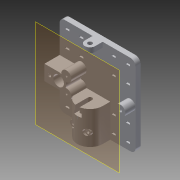
# Autodesk Inventor part: EFFECTOR SECONDARY PLATE
Saved by Autodesk Inventor 2013 (Build 170138000, 138)
## iProperties
Created: 2014-03-03
Part Number: EFFECTOR SECONDARY PLATE
Material: Generic
Document SubType Name: Modeling
Designer: employee
Density: 1 g/cm^3
Author: employee
Autodesk Inventor part; units mm, degrees
ref_plane "YZ Plane" through (0, 0, 0) normal (1, 0, 0) x (0, 1, 0)
ref_plane "XZ Plane" through (0, 0, 0) normal (0, 1, 0) x (-1, 0, 0)
ref_plane "XY Plane" through (0, 0, 0) normal (0, 0, 1) x (1, 0, 0)
sketch "Sketch1" plane through (0, 0, 0) normal (0, 0, 1) x (1, 0, 0)
  arc A0 (-32.5, 40) -> (-37.5, 35) centre (-32.5, 35) ccw projected
  line L0 (-37.5, 35) -> (-37.5, 12.5) projected
  arc A1 (-37.5, -35) -> (-32.5, -40) centre (-32.5, -35) ccw projected
  line L1 (-32.5, -40) -> (32.5, -40) projected
  arc A2 (32.5, -40) -> (37.5, -35) centre (32.5, -35) ccw projected
  line L2 (37.5, -35) -> (37.5, -12.5) projected
  arc A3 (37.5, 35) -> (32.5, 40) centre (32.5, 35) ccw projected
  line L3 (32.5, 40) -> (-32.5, 40) projected
  line L4 (-18, -34) -> (-18, -32.5) projected
  line L5 (-18, -32.5) -> (-14, -32.5) projected
  line L6 (-14, -32.5) -> (-14, -34) projected
  line L7 (-14, -34) -> (-18, -34) projected
  line L8 (-32, -16) -> (-28, -16) projected
  line L9 (-28, -16) -> (-28, -17.5) projected
  line L10 (-28, -17.5) -> (-32, -17.5) projected
  line L11 (-32, -17.5) -> (-32, -16) projected
  line L12 (-14, -16) -> (-14, -17.5) projected
  line L13 (-14, -17.5) -> (-18, -17.5) projected
  line L14 (-18, -17.5) -> (-18, -16) projected
  line L15 (-18, -16) -> (-14, -16) projected
  line L16 (-28, -34) -> (-32, -34) projected
  line L17 (-32, -34) -> (-32, -32.5) projected
  line L18 (-32, -32.5) -> (-28, -32.5) projected
  line L19 (-28, -32.5) -> (-28, -34) projected
  line L20 (18, -32.5) -> (18, -34) projected
  line L21 (18, -34) -> (14, -34) projected
  line L22 (14, -34) -> (14, -32.5) projected
  line L23 (14, -32.5) -> (18, -32.5) projected
  line L24 (28, -16) -> (32, -16) projected
  line L25 (32, -16) -> (32, -17.5) projected
  line L26 (32, -17.5) -> (28, -17.5) projected
  line L27 (28, -17.5) -> (28, -16) projected
  line L28 (14, -17.5) -> (14, -16) projected
  line L29 (14, -16) -> (18, -16) projected
  line L30 (18, -16) -> (18, -17.5) projected
  line L31 (18, -17.5) -> (14, -17.5) projected
  line L32 (32, -34) -> (28, -34) projected
  line L33 (28, -34) -> (28, -32.5) projected
  line L34 (28, -32.5) -> (32, -32.5) projected
  line L35 (32, -32.5) -> (32, -34) projected
  line L36 (-18, 32.5) -> (-18, 34) projected
  line L37 (-18, 34) -> (-14, 34) projected
  line L38 (-14, 34) -> (-14, 32.5) projected
  line L39 (-14, 32.5) -> (-18, 32.5) projected
  line L40 (-28, 16) -> (-32, 16) projected
  line L41 (-32, 16) -> (-32, 17.5) projected
  line L42 (-32, 17.5) -> (-28, 17.5) projected
  line L43 (-28, 17.5) -> (-28, 16) projected
  line L44 (-14, 17.5) -> (-14, 16) projected
  line L45 (-14, 16) -> (-18, 16) projected
  line L46 (-18, 16) -> (-18, 17.5) projected
  line L47 (-18, 17.5) -> (-14, 17.5) projected
  line L48 (-32, 34) -> (-28, 34) projected
  line L49 (-28, 34) -> (-28, 32.5) projected
  line L50 (-28, 32.5) -> (-32, 32.5) projected
  line L51 (-32, 32.5) -> (-32, 34) projected
  line L52 (14, 32.5) -> (14, 34) projected
  line L53 (14, 34) -> (18, 34) projected
  line L54 (18, 34) -> (18, 32.5) projected
  line L55 (18, 32.5) -> (14, 32.5) projected
  line L56 (28, 32.5) -> (28, 34) projected
  line L57 (28, 34) -> (32, 34) projected
  line L58 (32, 34) -> (32, 32.5) projected
  line L59 (32, 32.5) -> (28, 32.5) projected
  line L60 (18, 17.5) -> (18, 16) projected
  line L61 (18, 16) -> (14, 16) projected
  line L62 (14, 16) -> (14, 17.5) projected
  line L63 (14, 17.5) -> (18, 17.5) projected
  line L64 (32, 17.5) -> (32, 16) projected
  line L65 (32, 16) -> (28, 16) projected
  line L66 (28, 16) -> (28, 17.5) projected
  line L67 (28, 17.5) -> (32, 17.5) projected
  arc A4 (-32.5, -7.5) -> (-37.5, -12.5) centre (-32.5, -12.5) ccw projected
  line L68 (-37.5, -12.5) -> (-37.5, -35) projected
  arc A5 (37.5, -12.5) -> (32.5, -7.5) centre (32.5, -12.5) ccw projected
  line L69 (32.5, -7.5) -> (22.5, -7.5) projected
  arc A6 (22.5, 7.5) -> (22.5, -7.5) centre (22.5, 0) ccw projected
  line L70 (22.5, 7.5) -> (32.5, 7.5) projected
  arc A7 (32.5, 7.5) -> (37.5, 12.5) centre (32.5, 12.5) ccw projected
  line L71 (37.5, 12.5) -> (37.5, 35) projected
  arc A8 (-37.5, 12.5) -> (-32.5, 7.5) centre (-32.5, 12.5) ccw projected
  line L72 (-32.5, 7.5) -> (-22.5, 7.5) projected
  arc A9 (-22.5, -7.5) -> (-22.5, 7.5) centre (-22.5, 0) ccw projected
  line L73 (-22.5, -7.5) -> (-32.5, -7.5) projected
  point P0 (0, 0)
extrude "Extrusion1" add sketch "Sketch1" along normal blind 5
sketch "Sketch2" plane through (-32.5, -40, 0) normal (0, -1, 0) x (1, 0, 0)
  line L0 (65, 0) -> (0, 0) projected
  line L1 (0, 0) -> (0, 5) projected
  line L2 (20, 0) -> (20, 12.5)
  arc A0 (45, 12.5) -> (20, 12.5) centre (32.5, 12.5) ccw
  line L3 (45, 12.5) -> (45, 0)
  point P0 (32.5, 0)
  point P1 (32.5, 0)
  dimension "d2" = 12.5
  dimension "d3" = 12.5
  constraints: 4 end point, 2 point on circle, 2 point on line, 2 tangent, 1 centre point, 1 midpoint, 1 parallel, 1 perpendicular, 1 vertical alignment
  measures "d2" distance from line of A0.centre L0
  measures "d3" radius of A0
extrude "Extrusion2" add sketch "Sketch2" against normal blind 19
sketch "Sketch3" plane through (-32.5, -40, 0) normal (0, -1, 0) x (1, 0, 0)
  arc A0 (45, 12.5) -> (20, 12.5) centre (32.5, 12.5) ccw projected
  circle A1 centre (32.5, 12.5) radius 8.1
  point P0 (32.5, 0)
  dimension "d6" = 16.2
  constraints: 1 centre point, 1 coincident
  measures "d6" diameter of A1
extrude "Extrusion3" cut sketch "Sketch3" against normal up to surface (19 mm away)
sketch "Sketch4" plane through (0, 0, 0) normal (0, 0, -1) x (-1, 0, 0)
  line L0 (-32.5, -40) -> (32.5, -40) projected
  line L1 (-28, 17.5) -> (-28, 16) projected
  line L2 (-7.25, -27.5) -> (7.25, -27.5)
  circle A0 centre (-7.25, -27.5) radius 1.5
  circle A1 centre (7.25, -27.5) radius 1.5
  point P0 (0, 0)
  point P1 (0, -40)
  point P2 (0, -27.5)
  dimension "d10" = 12.5
  dimension "d11" = 3
  dimension "d12" = 14.5
  constraints: 2 centre point, 2 coincident, 2 end point, 2 midpoint, 1 equal radius, 1 perpendicular, 1 vertical alignment
  measures "d10" distance between parallel lines of L0 L2
  measures "d11" diameter of A1
  measures "d12" distance of L2.start L2.end
extrude "Extrusion4" cut sketch "Sketch4" against normal through all
ref_plane "Work Plane1" through (0, 0, 25) normal (0, 0, 1) x (1, 0, 0)
sketch "Sketch5" plane through (0, 0, 25) normal (0, 0, 1) x (1, 0, 0)
  circle A0 centre (7.25, -27.5) radius 1.5 projected
  circle A1 centre (-7.25, -27.5) radius 1.5 projected
  line L0 (32.5, -40) -> (-32.5, -40) projected
  arc A2 (-37.5, -35) -> (-32.5, -40) centre (-32.5, -35) ccw projected
  line L1 (-37.5, 12.5) -> (-37.5, 35) projected
  arc A3 (-32.5, 40) -> (-37.5, 35) centre (-32.5, 35) ccw projected
  line L2 (-32.5, 40) -> (32.5, 40) projected
  arc A4 (37.5, 35) -> (32.5, 40) centre (32.5, 35) ccw projected
  line L3 (37.5, -12.5) -> (37.5, -35) projected
  arc A5 (32.5, -40) -> (37.5, -35) centre (32.5, -35) ccw projected
  line L4 (-14, -32.5) -> (-18, -32.5) projected
  line L5 (-18, -32.5) -> (-18, -34) projected
  line L6 (-18, -34) -> (-14, -34) projected
  line L7 (-14, -34) -> (-14, -32.5) projected
  line L8 (-28, -17.5) -> (-28, -16) projected
  line L9 (-28, -16) -> (-32, -16) projected
  line L10 (-32, -16) -> (-32, -17.5) projected
  line L11 (-32, -17.5) -> (-28, -17.5) projected
  line L12 (-18, -17.5) -> (-14, -17.5) projected
  line L13 (-14, -17.5) -> (-14, -16) projected
  line L14 (-14, -16) -> (-18, -16) projected
  line L15 (-18, -16) -> (-18, -17.5) projected
  line L16 (-32, -32.5) -> (-32, -34) projected
  line L17 (-32, -34) -> (-28, -34) projected
  line L18 (-28, -34) -> (-28, -32.5) projected
  line L19 (-28, -32.5) -> (-32, -32.5) projected
  line L20 (14, -34) -> (18, -34) projected
  line L21 (18, -34) -> (18, -32.5) projected
  line L22 (18, -32.5) -> (14, -32.5) projected
  line L23 (14, -32.5) -> (14, -34) projected
  line L24 (32, -17.5) -> (32, -16) projected
  line L25 (32, -16) -> (28, -16) projected
  line L26 (28, -16) -> (28, -17.5) projected
  line L27 (28, -17.5) -> (32, -17.5) projected
  line L28 (18, -16) -> (14, -16) projected
  line L29 (14, -16) -> (14, -17.5) projected
  line L30 (14, -17.5) -> (18, -17.5) projected
  line L31 (18, -17.5) -> (18, -16) projected
  line L32 (28, -32.5) -> (28, -34) projected
  line L33 (28, -34) -> (32, -34) projected
  line L34 (32, -34) -> (32, -32.5) projected
  line L35 (32, -32.5) -> (28, -32.5) projected
  line L36 (-14, 34) -> (-18, 34) projected
  line L37 (-18, 34) -> (-18, 32.5) projected
  line L38 (-18, 32.5) -> (-14, 32.5) projected
  line L39 (-14, 32.5) -> (-14, 34) projected
  line L40 (-32, 17.5) -> (-32, 16) projected
  line L41 (-32, 16) -> (-28, 16) projected
  line L42 (-28, 16) -> (-28, 17.5) projected
  line L43 (-28, 17.5) -> (-32, 17.5) projected
  line L44 (-18, 16) -> (-14, 16) projected
  line L45 (-14, 16) -> (-14, 17.5) projected
  line L46 (-14, 17.5) -> (-18, 17.5) projected
  line L47 (-18, 17.5) -> (-18, 16) projected
  line L48 (-28, 32.5) -> (-28, 34) projected
  line L49 (-28, 34) -> (-32, 34) projected
  line L50 (-32, 34) -> (-32, 32.5) projected
  line L51 (-32, 32.5) -> (-28, 32.5) projected
  line L52 (18, 34) -> (14, 34) projected
  line L53 (14, 34) -> (14, 32.5) projected
  line L54 (14, 32.5) -> (18, 32.5) projected
  line L55 (18, 32.5) -> (18, 34) projected
  line L56 (32, 34) -> (28, 34) projected
  line L57 (28, 34) -> (28, 32.5) projected
  line L58 (28, 32.5) -> (32, 32.5) projected
  line L59 (32, 32.5) -> (32, 34) projected
  line L60 (14, 16) -> (18, 16) projected
  line L61 (18, 16) -> (18, 17.5) projected
  line L62 (18, 17.5) -> (14, 17.5) projected
  line L63 (14, 17.5) -> (14, 16) projected
  line L64 (28, 16) -> (32, 16) projected
  line L65 (32, 16) -> (32, 17.5) projected
  line L66 (32, 17.5) -> (28, 17.5) projected
  line L67 (28, 17.5) -> (28, 16) projected
  circle A6 centre (-7.25, -27.5) radius 3
  circle A7 centre (7.25, -27.5) radius 3
  line L68 (-37.5, -35) -> (-37.5, -12.5) projected
  arc A8 (-32.5, -7.5) -> (-37.5, -12.5) centre (-32.5, -12.5) ccw projected
  line L69 (-32.5, -7.5) -> (-22.5, -7.5) projected
  arc A9 (-22.5, -7.5) -> (-22.5, 7.5) centre (-22.5, 0) ccw projected
  line L70 (-22.5, 7.5) -> (-32.5, 7.5) projected
  arc A10 (-37.5, 12.5) -> (-32.5, 7.5) centre (-32.5, 12.5) ccw projected
  line L71 (37.5, 35) -> (37.5, 12.5) projected
  arc A11 (32.5, 7.5) -> (37.5, 12.5) centre (32.5, 12.5) ccw projected
  line L72 (32.5, 7.5) -> (22.5, 7.5) projected
  arc A12 (22.5, 7.5) -> (22.5, -7.5) centre (22.5, 0) ccw projected
  line L73 (22.5, -7.5) -> (32.5, -7.5) projected
  arc A13 (37.5, -12.5) -> (32.5, -7.5) centre (32.5, -12.5) ccw projected
  point P0 (0, 0)
  dimension "d16" = 6
  constraints: 2 centre point, 2 coincident, 1 equal radius
  measures "d16" diameter of A7
extrude "Extrusion5" add sketch "Sketch5" against normal up to surface contours A6 | A7
sketch "Sketch6" plane through (-7.25, -27.5, 25) normal (0, 0, 1) x (1, 0, 0)
  circle A0 centre (0, 0) radius 1.5 projected
  circle A1 centre (0, 0) radius 3 projected
  circle A2 centre (14.5, 0) radius 1.5 projected
  circle A3 centre (14.5, 0) radius 3 projected
  point P0 (7.25, 27.5)
extrude "Extrusion6" cut sketch "Sketch6" against normal blind 3
sketch "Sketch7" plane through (-32.5, -21, 0) normal (0, 1, 0) x (1, 0, 0)
  arc A0 (29.4406, -5) -> (35.5594, -5) centre (32.5, -12.5) ccw projected
  line L0 (20, -5) -> (29.4406, -5) projected
  line L1 (20, -5) -> (20, -12.5) projected
  arc A1 (20, -12.5) -> (45, -12.5) centre (32.5, -12.5) ccw projected
  line L2 (45, -12.5) -> (45, -5) projected
  line L3 (35.5594, -5) -> (45, -5) projected
  line L4 (29.4406, -5) -> (35.5594, -5)
  circle A2 centre (32.5, -12.5) radius 1
  point P0 (32.5, 0)
  dimension "d22" = 2
  constraints: 2 end point, 1 centre point, 1 coincident, 1 collinear
  measures "d22" diameter of A2
extrude "Extrusion7" add sketch "Sketch7" along normal blind 5
fillet "Fillet1" radius 2 1 edges at (-1, -16, 12.5)
sketch "Sketch8" plane through (-32.5, -16, 0) normal (0, 1, 0) x (1, 0, 0)
  line L0 (20, -5) -> (45, -5) projected
  line L1 (20, -5) -> (20, -12.5) projected
  arc A0 (20, -12.5) -> (45, -12.5) centre (32.5, -12.5) ccw projected
  line L2 (45, -12.5) -> (45, -5) projected
  circle A1 centre (32.5, -12.5) radius 3 projected
  line L3 (32.5, -8.3431) -> (36.1, -10.4215)
  line L4 (36.1, -10.4215) -> (36.1, -14.5785)
  line L5 (36.1, -14.5785) -> (32.5, -16.6569)
  line L6 (32.5, -16.6569) -> (28.9, -14.5785)
  line L7 (28.9, -14.5785) -> (28.9, -10.4215)
  line L8 (28.9, -10.4215) -> (32.5, -8.3431)
  line L9 (28.9, -14.5785) -> (28.9, -24.4704)
  line L10 (36.1, -14.5785) -> (36.1, -24.4704)
  point P0 (32.5, 0)
  dimension "d28" = 7.2
  constraints: 16 end point, 2 point on circle, 1 coincident, 1 collinear, 1 parallel, 1 vertical, 13 other
  measures "d28" distance between parallel lines of L4 L7
extrude "Extrusion8" add sketch "Sketch8" along normal blind 3.5 contours L0 L2 A0 L10 L4 L3 L8 L7 L9 L1
sketch "Sketch9" plane through (-32.5, -12.5, 0) normal (0, 1, 0) x (1, 0, 0)
  line L0 (20, -5) -> (45, -5) projected
  line L1 (20, -5) -> (20, -12.5) projected
  arc A0 (20, -12.5) -> (28.9, -24.4704) centre (32.5, -12.5) ccw projected
  arc A1 (36.1, -24.4704) -> (45, -12.5) centre (32.5, -12.5) ccw projected
  line L2 (45, -12.5) -> (45, -5) projected
  line L3 (30.4, -24.8212) -> (30.4, -12.5)
  arc A2 (34.6, -12.5) -> (30.4, -12.5) centre (32.5, -12.5) ccw
  line L4 (34.6, -12.5) -> (34.6, -24.8233)
  arc A3 (28.9, -24.4704) -> (30.4, -24.8212) centre (32.4911, -12.4973) ccw
  arc A4 (34.6, -24.8233) -> (36.1, -24.4704) centre (32.4911, -12.4973) ccw
  point P0 (32.5, 0)
  dimension "d31" = 2.1
  constraints: 7 point on circle, 4 end point, 3 centre point, 2 parallel, 2 tangent, 1 coincident
  measures "d31" radius of A2
extrude "Extrusion9" add sketch "Sketch9" along normal blind 5
sketch "Sketch10" plane through (-32.5, 40, 0) normal (0, 1, 0) x (1, 0, 0)
  line L0 (65, -5) -> (0, -5) projected
  line L1 (65, 0) -> (65, -5) projected
  arc A0 (34.6, -12.5) -> (30.4, -12.5) centre (32.5, -12.5) ccw projected
  line L2 (27.5, -5) -> (27.5, -12.5)
  arc A1 (27.5, -12.5) -> (37.5, -12.5) centre (32.5, -12.5) ccw
  line L3 (37.5, -12.5) -> (37.5, -5)
  circle A2 centre (32.5, -12.5) radius 2.1
  point P0 (32.5, 0)
  dimension "d35" = 5
  constraints: 4 end point, 2 point on circle, 2 point on line, 2 tangent, 1 centre point, 1 coincident, 1 concentric, 1 horizontal alignment, 1 parallel, 1 perpendicular, 2 other
  measures "d35" radius of A1
extrude "Extrusion10" add sketch "Sketch10" against normal blind 5
sketch "Sketch11" plane through (0, 0, 5) normal (0, 0, 1) x (1, 0, 0)
  line L0 (-37.5, 35) -> (-37.5, -35) projected
  line L1 (32, 17.5) -> (32, 16) projected
  line L2 (-37.5, 7.5) -> (-23.5, 7.5)
  arc A0 (-23.5, -7.5) -> (-23.5, 7.5) centre (-23.5, 0) ccw
  line L3 (-23.5, -7.5) -> (-37.5, -7.5)
  point P0 (0, 0)
  dimension "d40" = 7.5
  dimension "d42" = 14
  constraints: 4 end point, 2 perpendicular, 2 point on circle, 2 point on line, 2 tangent, 1 centre point, 1 horizontal alignment
  measures "d40" radius of A0
  measures "d42" distance of L2.start L2.end
extrude "Extrusion11" add sketch "Sketch11" along normal blind 15
sketch "Sketch12" plane through (0, 0, 0) normal (0, 0, -1) x (-1, 0, 0)
  arc A0 (37.5, -12.5) -> (32.5, -7.5) centre (32.5, -12.5) ccw projected
  line L0 (32.5, -7.5) -> (22.5, -7.5) projected
  arc A1 (22.5, 7.5) -> (22.5, -7.5) centre (22.5, 0) ccw projected
  line L1 (22.5, 7.5) -> (32.5, 7.5) projected
  arc A2 (32.5, 7.5) -> (37.5, 12.5) centre (32.5, 12.5) ccw projected
  arc A3 (-37.5, 12.5) -> (-32.5, 7.5) centre (-32.5, 12.5) ccw projected
  line L2 (-32.5, 7.5) -> (-22.5, 7.5) projected
  arc A4 (-22.5, -7.5) -> (-22.5, 7.5) centre (-22.5, 0) ccw projected
  line L3 (-22.5, -7.5) -> (-32.5, -7.5) projected
  arc A5 (-32.5, -7.5) -> (-37.5, -12.5) centre (-32.5, -12.5) ccw projected
  line L4 (-28, 17.5) -> (-28, 16) projected
  line L5 (-37.5, 12.5) -> (-37.5, -12.5)
  line L6 (37.5, -12.5) -> (37.5, 12.5)
  point P0 (0, 0)
  constraints: 4 end point, 3 tangent, 2 parallel, 1 point on circle
extrude "Extrusion12" add sketch "Sketch12" against normal up to surface (5 mm away)
sketch "Sketch13" plane through (0, 0, 20) normal (0, 0, 1) x (1, 0, 0)
  circle A0 centre (-15.8668, -7.6332) radius 1.125 projected
  circle A1 centre (-15.8668, -7.6332) radius 5
  point P0 (0, 0)
  dimension "d47" = 10
  constraints: 1 centre point, 1 coincident
  measures "d47" diameter of A1
extrude "Extrusion13" add sketch "Sketch13" against normal up to surface (15 mm away) contours A0 | A1
mirror "Mirror1" about plane through (0, 0, 0) normal (0, 1, 0) of "Extrusion13"
sketch "Sketch14" plane through (0, 0, 20) normal (0, 0, 1) x (1, 0, 0)
  arc A0 (-20.8275, -7.0077) -> (-16.4923, -2.6725) centre (-15.8668, -7.6332) ccw projected
  arc A1 (-16.4923, 2.6725) -> (-20.8275, 7.0077) centre (-15.8668, 7.6332) ccw projected
  circle A2 centre (-15.8668, 7.6332) radius 1
  circle A3 centre (-15.8668, -7.6332) radius 1
  point P0 (-11.2662, -5.675)
  point P1 (-14.0758, -2.965)
  point P2 (-14.0758, 2.965)
  point P3 (-20.535, 9.4242)
  point P4 (0, 0)
  dimension "d55" = 2
  constraints: 2 centre point, 2 coincident, 1 equal radius
  measures "d55" diameter of A2
extrude "Extrusion14" cut sketch "Sketch14" against normal through all
sketch "Sketch15" plane through (0, 0, 20) normal (0, 0, 1) x (1, 0, 0)
  arc A0 (-16.4923, -2.6725) -> (-16.4923, 2.6725) centre (-23.5, 0) ccw projected
  circle A1 centre (-23.5, 0) radius 5.25
  point P0 (0, 0)
  dimension "d59" = 10.5
  constraints: 1 centre point, 1 coincident
  measures "d59" diameter of A1
extrude "Extrusion15" cut sketch "Sketch15" against normal blind 10.5
sketch "Sketch16" plane through (-23.5, 0, 9.5) normal (0, 0, 1) x (1, 0, 0)
  circle A0 centre (0, 0) radius 5.25 projected
  circle A1 centre (0, 0) radius 3.25
  point P0 (23.5, 0)
  dimension "d63" = 6.5
  constraints: 1 centre point, 1 coincident
  measures "d63" diameter of A1
extrude "Extrusion16" cut sketch "Sketch16" against normal through all contours A1
sketch "Sketch17" plane through (0, 0, 0) normal (0, 0, -1) x (-1, 0, 0)
  line L0 (37.5, -35) -> (37.5, 35) projected
  circle A0 centre (32.5, 0) radius 3
  circle A1 centre (32.5, 0) radius 1.5
  point P0 (0, 0)
  dimension "d68" = 6
  dimension "d70" = 3
  dimension "d71" = 5
  constraints: 2 centre point, 1 coincident
  measures "d68" diameter of A0
  measures "d70" diameter of A1
  measures "d71" distance from line of L0 A1.centre
extrude "Extrusion17" cut sketch "Sketch17" against normal through all contours A1
sketch "Sketch18" plane through (0, 0, 0) normal (0, 0, -1) x (-1, 0, 0)
  line L0 (-37.5, 35) -> (-37.5, -35) projected
  circle A0 centre (-32.5, 0) radius 1.5
  point P0 (0, 0)
  point P1 (-37.5, 0)
  dimension "d74" = 3
  dimension "d76" = 5
  constraints: 1 centre point, 1 horizontal alignment, 1 midpoint
  measures "d74" diameter of A0
  measures "d76" distance from line of A0.centre L0
extrude "Extrusion18" cut sketch "Sketch18" against normal through all
sketch "Sketch19" plane through (0, 0, 5) normal (0, 0, 1) x (1, 0, 0)
  circle A0 centre (32.5, 0) radius 1.5 projected
  line L0 (37.5, -35) -> (37.5, 35) projected
  circle A1 centre (32.5, 0) radius 5
  point P0 (0, 0)
  constraints: 1 centre point, 1 coincident, 1 tangent
extrude "Extrusion19" add sketch "Sketch19" along normal blind 10
body "Solid1"
